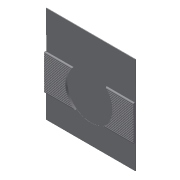
# Autodesk Inventor part: 00_chip_01_old
Saved by Autodesk Inventor 2019.4 (Build 234330000, 330)
## iProperties
Created: 2020-05-10
Part Number: 00_chip_01_old
Material: Generic
Document SubType Name: Modeling
Designer: diederichbenedict
Density: 1 g/cm^3
Appearance: Default
Mass: 0.49382 g
Surface Area: 15.5676 cm^2
Volume: 0.49382 cm^3
Author: diederichbenedict
Autodesk Inventor part; units mm, degrees
ref_plane "YZ Plane" through (0, 0, 0) normal (1, 0, 0) x (0, 1, 0)
ref_plane "XZ Plane" through (0, 0, 0) normal (0, 1, 0) x (-1, 0, 0)
ref_plane "XY Plane" through (0, 0, 0) normal (0, 0, 1) x (1, 0, 0)
sketch "Sketch1" plane through (0, 0, 0) normal (0, 0, 1) x (1, 0, 0)
  line L0 (0, 0) -> (24, 0)
  line L1 (24, 0) -> (24, 26)
  line L2 (24, 26) -> (0, 26)
  line L3 (0, 26) -> (0, 0)
  dimension "d0" = 24
  dimension "d1" = 26
  constraints: 8 end point, 2 parallel, 1 horizontal, 1 perpendicular
  measures "d0" distance of L2.end L1.end
  measures "d1" distance of L1.end L0.end
extrude "Extrusion1" add sketch "Sketch1" along normal blind 0.17
sketch "Sketch2" plane through (0, 0, 0.17) normal (0, 0, 1) x (1, 0, 0)
  line L0 (0, 0) -> (24, 0) projected
  line L1 (24, 0) -> (24, 26) projected
  line L2 (24, 26) -> (0, 26) projected
  line L3 (0, 26) -> (0, 0) projected
  line L4 (24, 0) -> (24, 26) projected
  line L5 (0, 19.73) -> (24, 19.73)
  line L6 (24, 19.73) -> (24, 10.73)
  line L7 (24, 10.73) -> (0, 10.73)
  line L8 (0, 10.73) -> (0, 19.73)
  dimension "d4" = 9
  dimension "d5" = 6.27
  constraints: 8 end point, 2 parallel, 2 point on line, 1 horizontal, 1 perpendicular
  measures "d4" distance of L5.end L6.end
  measures "d5" distance between parallel lines of L5 L2
extrude "Extrusion2" cut sketch "Sketch2" against normal blind 0.05 contours L3 L5 L1 L7
sketch "Sketch3" plane through (24, 0, 0) normal (1, 0, 0) x (0, 0, -1)
  line L0 (-0.17, 0) -> (-0.17, 10.73) projected
  line L1 (0, 0) -> (-0.17, 0) projected
  line L2 (0, 0) -> (0, 26) projected
  line L3 (0, 26) -> (-0.17, 26) projected
  circle A0 centre (-0.42, 15.7925) radius 0.3
  line L4 (-0.12, 19.73) -> (-0.12, 10.73) projected
  line L5 (-0.12, 10.73) -> (-0.17, 10.73) projected
  line L6 (-0.17, 19.73) -> (-0.17, 26) projected
  line L7 (-0.17, 19.73) -> (-0.12, 19.73) projected
  line L8 (-0.12, 19.73) -> (-0.12, 10.73) projected
  constraints: 1 centre point, 1 tangent
extrude "Extrusion3" add sketch "Sketch3" against normal up to surface (24 mm away) contours A0
pattern_linear "Rectangular Pattern1" count 24 spacing 0.39 along (0, -1, 0) of "Extrusion3"
sketch "Sketch5" plane through (0, 0, 0.12) normal (0, 0, 1) x (1, 0, 0)
  ellipse E0 centre (12.6795, 11.6125) end of major axis (0.2295, 11.6125) minor radius 11.5023 construction
  circle A0 centre (12.6795, 11.6125) radius 13 construction
  line L0 (24, 26) -> (0, 26) construction
  line L1 (0, 0) -> (24, 0) construction
  line L2 (24, 0) -> (24, 6.6567) construction
  line L3 (0, 6.6567) -> (0, 0) construction
  line L4 (24, 26) -> (0, 0) construction
  line L5 (0, 26) -> (24, 0) construction
  circle A1 centre (12, 11.6125) radius 6.3157
  constraints: 4 end point, 1 centre point, 1 other
extrude "Extrusion5" cut sketch "Sketch5" along normal blind 10
body "Solid1"
